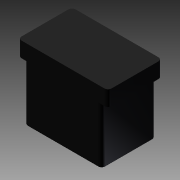
# Autodesk Inventor part: battery
Saved by Autodesk Inventor 2012 (Build 160160000, 160)
## iProperties
Created: 2012-03-08
Part Number: battery
Material: Default
Document SubType Name: Modeling
Designer: esv
Mass: 21545.6 g
Surface Area: 3513.22 cm^2
Volume: 13467.3 cm^3
Density: 1.59985 g/cm^3
Author: esv
Autodesk Inventor part; units mm, degrees
ref_plane "YZ Plane" through (0, 0, 0) normal (1, 0, 0) x (0, 1, 0)
ref_plane "XZ Plane" through (0, 0, 0) normal (0, 1, 0) x (-1, 0, 0)
ref_plane "XY Plane" through (0, 0, 0) normal (0, 0, 1) x (1, 0, 0)
sketch "Sketch1" plane through (0, 0, 0) normal (0, 0, 1) x (1, 0, 0)
  line L0 (-136.525, 0) -> (136.525, 0)
  line L1 (136.525, 0) -> (136.525, 196.85)
  line L2 (136.525, 196.85) -> (-136.525, 196.85)
  line L3 (-136.525, 196.85) -> (-136.525, 0)
  line L4 (-158.75, 196.85) -> (158.75, 196.85)
  line L5 (158.75, 196.85) -> (158.75, 250.825)
  line L6 (158.75, 250.825) -> (-158.75, 250.825)
  line L7 (-158.75, 250.825) -> (-158.75, 196.85)
  point P0 (0, 0)
  point P1 (0, 196.85)
  point P2 (0, 0)
  dimension "d0" = 250.825
  dimension "d1" = 317.5
  dimension "d2" = 196.85
  dimension "d3" = 273.05
  constraints: 16 end point, 4 parallel, 3 midpoint, 2 horizontal, 2 perpendicular, 1 coincident, 1 point on line
  measures "d0" distance between parallel lines of L0 L6
  measures "d1" distance between parallel lines of L5 L7
  measures "d2" distance of L2.end L0.start
  measures "d3" distance of L0.start L0.end
extrude "Extrusion1" add sketch "Sketch1" along normal blind 190.5
fillet "Fillet1" radius 3.175 4 edges at (0, 0, 190.5) (136.525, 0, 95.25) (0, 0, 0) (-136.525, 0, 95.25)
fillet "Fillet1" radius 12.7 8 edges at (136.525, 98.425, 190.5) (136.525, 98.425, 0) (-136.525, 98.425, 190.5) (-136.525, 98.425, 0) (-158.75, 223.8375, 190.5) (-158.75, 223.8375, 0) (158.75, 223.8375, 190.5) (158.75, 223.8375, 0)
body "Solid1"
